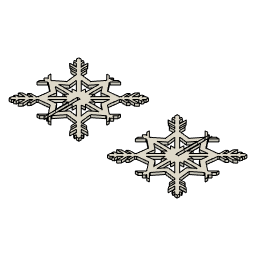
fulg (Autodesk Fusion 360 design; units mm, degrees)
Autodesk Fusion 360 part; units mm, degrees
sketch "Sketch1" plane through (0, 0, 0) normal (0, 1, 0) x (1, 0, 0)
  line L0 (40, 40) -> (-40, 40) construction
  line L1 (-40, 40) -> (-40, -40) construction
  line L2 (-40, -40) -> (40, -40) construction
  line L3 (40, -40) -> (40, 40) construction
  line L4 (40, 40) -> (-40, -40) construction
  dimension "d1" = 80
  dimension "d2" = 80
  constraint perpendicular L0 L1
  constraint parallel L0 L2
  constraint parallel L1 L3
  constraint horizontal L0
  constraint coincident L4 origin
  measures "d1" distance of L1.end L2.end
  measures "d2" distance of L0.end L1.end
sketch "Sketch3" plane through (0, 0, 0) normal (0, 1, 0) x (1, 0, 0)
  line L0 (0, 40) -> (0, 35) construction
  line L1 (40, 0) -> (46.0201, 0) construction
  line L2 (-40, 0) -> (-46.178, 0) construction
  line L3 (0.0024, 40) -> (-0.0024, 40)
  arc A0 (0.0024, 40) -> (-0.0024, 40) centre (0, 37.5) ccw
  line L4 (-40, 40) -> (-40, 37.1716)
  line L5 (-40, 40) -> (-37.1716, 40)
  line L6 (40, -40) -> (40, -37.1716)
  line L7 (40, -37.1716) -> (40, -40)
  line L8 (37.1716, -40) -> (40, -40)
  line L9 (-40, -40) -> (-38, -40) construction
  line L10 (-40, -40) -> (-40, -37.1716)
  line L11 (-40, -40) -> (-37.1716, -40)
  line L12 (40, 40) -> (40, 37.1716)
  line L13 (40, 40) -> (37.1716, 40)
  line L14 (-5.3576, 12.9343) -> (-5.514, 8.3424)
  line L15 (-5.3576, 12.9343) -> (-2, 9.798)
  line L16 (12.9343, -5.3576) -> (8.3424, -5.514)
  line L17 (12.9343, -5.3576) -> (9.798, -2)
  line L18 (5.3576, 12.9343) -> (5.514, 8.3424)
  line L19 (5.3576, 12.9343) -> (2, 9.798)
  line L20 (-5.3576, -12.9343) -> (-5.514, -8.3424)
  line L21 (-5.3576, -12.9343) -> (-2, -9.798)
  line L22 (-12.9343, 5.3576) -> (-8.3424, 5.514)
  line L23 (-12.9343, 5.3576) -> (-9.798, 2)
  line L24 (-12.9343, -5.3576) -> (-9.798, -2)
  line L25 (-12.9343, -5.3576) -> (-8.3424, -5.514)
  line L26 (5.3576, -12.9343) -> (5.514, -8.3424)
  line L27 (5.3576, -12.9343) -> (2, -9.798)
  line L28 (12.9343, 5.3576) -> (9.798, 2)
  line L29 (12.9343, 5.3576) -> (8.3424, 5.514)
  line L30 (-16.2068, 19.0352) -> (-5.514, 8.3424)
  line L31 (-7.4559, 17.9962) -> (-2, 24.899)
  line L32 (-2, 24.899) -> (-2, 9.798)
  line L33 (-7.4559, 17.9962) -> (-16.2068, 19.0352)
  line L34 (-19.0352, 16.2068) -> (-8.3424, 5.514)
  line L35 (-24.899, -2) -> (-9.798, -2)
  line L36 (-8.3424, -5.514) -> (-19.0352, -16.2068)
  line L37 (-16.2068, -19.0352) -> (-5.514, -8.3424)
  line L38 (-2, -9.798) -> (-2, -24.899)
  line L39 (2, -24.899) -> (2, -9.798)
  line L40 (5.514, -8.3424) -> (16.2068, -19.0352)
  line L41 (19.0352, -16.2068) -> (8.3424, -5.514)
  line L42 (9.798, -2) -> (24.899, -2)
  line L43 (24.899, 2) -> (9.798, 2)
  line L44 (8.3424, 5.514) -> (19.0352, 16.2068)
  line L45 (16.2068, 19.0352) -> (5.514, 8.3424)
  line L46 (2, 24.899) -> (2, 9.798)
  line L47 (7.4559, 17.9962) -> (16.2068, 19.0352)
  line L48 (7.4559, 17.9962) -> (2, 24.899)
  line L49 (17.9962, 7.4559) -> (24.899, 2)
  line L50 (17.9962, 7.4559) -> (19.0352, 16.2068)
  line L51 (17.9962, -7.4559) -> (19.0352, -16.2068)
  line L52 (24.899, -2) -> (17.9962, -7.4559)
  line L53 (7.4559, -17.9962) -> (2, -24.899)
  line L54 (7.4559, -17.9962) -> (16.2068, -19.0352)
  line L55 (-7.4559, -17.9962) -> (-16.2068, -19.0352)
  line L56 (-7.4559, -17.9962) -> (-2, -24.899)
  line L57 (-17.9962, -7.4559) -> (-24.899, -2)
  line L58 (-17.9962, -7.4559) -> (-19.0352, -16.2068)
  line L59 (-17.9962, 7.4559) -> (-19.0352, 16.2068)
  line L60 (-17.9962, 7.4559) -> (-24.899, 2)
  line L61 (-23.2912, 9.644) -> (-27.9994, 5.9227)
  line L62 (-23.2912, 9.644) -> (-24.0004, 15.6173)
  line L63 (-24.0004, 15.6173) -> (-24.7487, 21.9203)
  line L64 (-23.2912, 9.644) -> (-32.9624, 2)
  line L65 (-24.9199, 2) -> (-9.798, 2)
  line L66 (23.2912, 9.644) -> (32.9624, 2)
  line L67 (23.2912, 9.644) -> (24.7487, 21.9203)
  line L68 (19.0352, 16.2068) -> (8.3424, 5.514)
  line L69 (9.798, 2) -> (24.9199, 2)
  line L70 (23.2912, -9.644) -> (24.0004, -15.6173)
  line L71 (32.9624, -2) -> (23.2912, -9.644)
  line L72 (23.2912, -9.644) -> (24.7487, -21.9203)
  line L73 (9.644, -23.2912) -> (15.6173, -24.0004)
  line L74 (9.644, -23.2912) -> (2, -32.9624)
  line L75 (9.644, -23.2912) -> (21.9203, -24.7487)
  line L76 (7, -9.8284) -> (7, -9.798)
  line L77 (-9.644, -23.2912) -> (-7, -26.6364)
  line L78 (-9.644, -23.2912) -> (-15.6173, -24.0004)
  line L79 (-9.644, -23.2912) -> (-2, -32.9624)
  line L80 (-9.644, -23.2912) -> (-21.9203, -24.7487)
  line L81 (-23.2912, -9.644) -> (-26.6364, -7)
  line L82 (-23.2912, -9.644) -> (-24.0004, -15.6173)
  line L83 (-23.2912, -9.644) -> (-32.9624, -2)
  line L84 (-23.2912, -9.644) -> (-24.7487, -21.9203)
  line L85 (3, 10.7321) -> (3, 9.798)
  line L86 (-9.644, 23.2912) -> (-15.6173, 24.0004)
  line L87 (-9.644, 23.2912) -> (-2, 32.9624)
  line L88 (-9.644, 23.2912) -> (-21.9203, 24.7487)
  line L89 (9.644, 23.2912) -> (15.6173, 24.0004)
  line L90 (9.644, 23.2912) -> (7, 26.6364)
  line L91 (-7, 9.8284) -> (-7, 9.798)
  line L92 (9.644, 23.2912) -> (2, 32.9624)
  line L93 (9.644, 23.2912) -> (21.9203, 24.7487)
  line L94 (5.514, 8.3424) -> (16.2068, 19.0352)
  line L95 (2, 9.798) -> (2, 24.9199)
  line L96 (-2, 24.9199) -> (-2, 9.798)
  line L97 (-5.514, 8.3424) -> (-16.2068, 19.0352)
  line L98 (-9.798, -2) -> (-24.9199, -2)
  line L99 (-5.514, -8.3424) -> (-16.2068, -19.0352)
  line L100 (-2, -9.798) -> (-2, -24.9199)
  line L101 (2, -24.9199) -> (2, -9.798)
  line L102 (5.514, -8.3424) -> (16.2068, -19.0352)
  line L103 (19.0352, -16.2068) -> (8.3424, -5.514)
  line L104 (24.9199, -2) -> (9.798, -2)
  line L105 (-40, 0) -> (-38, 2)
  line L106 (-40, 0) -> (-38, -2)
  line L107 (-34, 2) -> (-40, 8)
  line L108 (-37, 2) -> (-40, 5)
  line L109 (-40, 5) -> (-40, 8)
  line L110 (-37, -2) -> (-40, -5)
  line L111 (-40, -5) -> (-40, -8)
  line L112 (-40, -8) -> (-34, -2)
  line L113 (-38, 2) -> (-37, 2)
  line L114 (-34, 2) -> (-32.9624, 2)
  line L115 (-32.9624, -2) -> (-34, -2)
  line L116 (-37, -2) -> (-38, -2)
  line L117 (40, 0) -> (37.9962, 2)
  line L118 (40, 0) -> (38.0038, -2)
  line L119 (37.0369, 2) -> (40, 4.9687)
  line L120 (40, 4.9687) -> (40, 7.9488)
  line L121 (40, 7.9488) -> (34.0625, 2)
  line L122 (37.0369, -2) -> (40, -4.9575)
  line L123 (40, -4.9575) -> (40, -8)
  line L124 (40, -8) -> (33.9886, -2)
  line L125 (32.9624, 2) -> (34.0625, 2)
  line L126 (37.0369, 2) -> (37.9962, 2)
  line L127 (38.0038, -2) -> (37.0369, -2)
  line L128 (33.9886, -2) -> (32.9624, -2)
  line L129 (0, -40) -> (2, -38)
  line L130 (0, -40) -> (-2, -38)
  line L131 (-2, -36.9976) -> (-5.0024, -40)
  line L132 (-5.0024, -40) -> (-7.9912, -40)
  line L133 (-7.9912, -40) -> (-2, -34.0088)
  line L134 (2, -34.0088) -> (7.9912, -40)
  line L135 (7.9912, -40) -> (4.9956, -40)
  line L136 (4.9956, -40) -> (2, -37.0044)
  line L137 (2, -38) -> (2, -37.0044)
  line L138 (2, -34.0088) -> (2, -32.9624)
  line L139 (-2, -32.9624) -> (-2, -34.0088)
  line L140 (-2, -36.9976) -> (-2, -38)
  line L141 (-0.0024, 40) -> (2, 38)
  line L142 (-0.0024, 40) -> (-2, 38)
  line L143 (-2, 36.9767) -> (-5.027, 40)
  line L144 (-5.027, 40) -> (-7.9448, 40)
  line L145 (-7.9448, 40) -> (-2, 34.0624)
  line L146 (2, 37) -> (4.9963, 40)
  line L147 (4.9963, 40) -> (8, 40)
  line L148 (8, 40) -> (2, 33.9927)
  line L149 (2, 32.9624) -> (2, 33.9927)
  line L150 (2, 37) -> (2, 38)
  line L151 (-2, 38) -> (-2, 36.9767)
  line L152 (-2, 34.0624) -> (-2, 32.9624)
  line L153 (-35.01, 37.8385) -> (-35.01, 40)
  line L154 (-35.01, 40) -> (-32.9636, 38.9192)
  line L155 (-32.9636, 38.9192) -> (-32.9636, 35.792)
  line L156 (-37.8689, 35.0405) -> (-40, 35.0405)
  line L157 (-40, 35.0405) -> (-38.9345, 32.942)
  line L158 (-38.9345, 32.942) -> (-35.7705, 32.942)
  line L159 (-29.5459, 32.3743) -> (-29.5459, 40)
  line L160 (-29.5459, 40) -> (-27, 37)
  line L161 (-27, 37) -> (-27, 29.8284)
  line L162 (-32.3743, 29.5459) -> (-40, 29.5459)
  line L163 (-40, 29.5459) -> (-37, 27)
  line L164 (-37, 27) -> (-29.8284, 27)
  line L165 (-22.999, 25.8274) -> (-22.999, 32)
  line L166 (-22.999, 32) -> (-24.9897, 33.9907)
  line L167 (-24.9897, 33.9907) -> (-24.9897, 27.8181)
  line L168 (-25.7878, 22.9594) -> (-32, 22.9594)
  line L169 (-32, 22.9594) -> (-34.0154, 24.9748)
  line L170 (-34.0154, 24.9748) -> (-27.8032, 24.9748)
  line L171 (-40, 37.1716) -> (-37.8689, 35.0405)
  line L172 (-35.01, 37.8385) -> (-37.1716, 40)
  line L173 (-29.5459, 32.3743) -> (-32.9636, 35.792)
  line L174 (-21.9203, 24.7487) -> (-22.999, 25.8274)
  line L175 (-24.9897, 27.8181) -> (-27, 29.8284)
  line L176 (-25.7878, 22.9594) -> (-24.7487, 21.9203)
  line L177 (-35.7705, 32.942) -> (-32.3743, 29.5459)
  line L178 (-29.8284, 27) -> (-27.8032, 24.9748)
  line L179 (35.01, 37.8385) -> (35.01, 40)
  line L180 (35.01, 40) -> (32.9636, 38.9192)
  line L181 (32.9636, 38.9192) -> (32.9636, 35.792)
  line L182 (37.8689, 35.0405) -> (40, 35.0405)
  line L183 (40, 35.0405) -> (38.9345, 32.942)
  line L184 (38.9345, 32.942) -> (35.7705, 32.942)
  line L185 (32.3743, 29.5459) -> (40, 29.5459)
  line L186 (40, 29.5459) -> (37, 27)
  line L187 (37, 27) -> (29.8284, 27)
  line L188 (34.0154, 24.9748) -> (27.8032, 24.9748)
  line L189 (32, 22.9594) -> (34.0154, 24.9748)
  line L190 (25.7878, 22.9594) -> (32, 22.9594)
  line L191 (24.9897, 33.9907) -> (24.9897, 27.8181)
  line L192 (22.999, 32) -> (24.9897, 33.9907)
  line L193 (22.999, 25.8274) -> (22.999, 32)
  line L194 (27, 37) -> (27, 29.8284)
  line L195 (29.5459, 40) -> (27, 37)
  line L196 (29.5459, 32.3743) -> (29.5459, 40)
  line L197 (32.9636, -38.9192) -> (32.9636, -35.792)
  line L198 (35.01, -40) -> (32.9636, -38.9192)
  line L199 (35.01, -37.8385) -> (35.01, -40)
  line L200 (29.5459, -32.3743) -> (29.5459, -40)
  line L201 (29.5459, -40) -> (27, -37)
  line L202 (27, -37) -> (27, -29.8284)
  line L203 (24.9897, -33.9907) -> (24.9897, -27.8181)
  line L204 (22.999, -32) -> (24.9897, -33.9907)
  line L205 (22.999, -25.8274) -> (22.999, -32)
  line L206 (34.0154, -24.9748) -> (27.8032, -24.9748)
  line L207 (25.7878, -22.9594) -> (32, -22.9594)
  line L208 (32, -22.9594) -> (34.0154, -24.9748)
  line L209 (37, -27) -> (29.8284, -27)
  line L210 (40, -29.5459) -> (37, -27)
  line L211 (32.3743, -29.5459) -> (40, -29.5459)
  line L212 (38.9345, -32.942) -> (35.7705, -32.942)
  line L213 (40, -35.0405) -> (38.9345, -32.942)
  line L214 (37.8689, -35.0405) -> (40, -35.0405)
  line L215 (-22.999, -25.8274) -> (-22.999, -32)
  line L216 (-22.999, -32) -> (-24.9897, -33.9907)
  line L217 (-24.9897, -33.9907) -> (-24.9897, -27.8181)
  line L218 (-27, -37) -> (-27, -29.8284)
  line L219 (-29.5459, -40) -> (-27, -37)
  line L220 (-29.5459, -32.3743) -> (-29.5459, -40)
  line L221 (-32.9636, -38.9192) -> (-32.9636, -35.792)
  line L222 (-35.01, -40) -> (-32.9636, -38.9192)
  line L223 (-35.01, -37.8385) -> (-35.01, -40)
  line L224 (-37.8689, -35.0405) -> (-40, -35.0405)
  line L225 (-40, -35.0405) -> (-38.9345, -32.942)
  line L226 (-38.9345, -32.942) -> (-35.7705, -32.942)
  line L227 (-32.3743, -29.5459) -> (-40, -29.5459)
  line L228 (-40, -29.5459) -> (-37, -27)
  line L229 (-37, -27) -> (-29.8284, -27)
  line L230 (-34.0154, -24.9748) -> (-27.8032, -24.9748)
  line L231 (-32, -22.9594) -> (-34.0154, -24.9748)
  line L232 (-25.7878, -22.9594) -> (-32, -22.9594)
  line L233 (-25.7878, -22.9594) -> (-24.7487, -21.9203)
  line L234 (-29.8284, -27) -> (-27.8032, -24.9748)
  line L235 (-40, -37.1716) -> (-37.8689, -35.0405)
  line L236 (-35.7705, -32.942) -> (-32.3743, -29.5459)
  line L237 (-35.01, -37.8385) -> (-37.1716, -40)
  line L238 (-29.5459, -32.3743) -> (-32.9636, -35.792)
  line L239 (-21.9203, -24.7487) -> (-22.999, -25.8274)
  line L240 (-24.9897, -27.8181) -> (-27, -29.8284)
  line L241 (21.9203, -24.7487) -> (22.999, -25.8274)
  line L242 (24.9897, -27.8181) -> (27, -29.8284)
  line L243 (29.5459, -32.3743) -> (32.9636, -35.792)
  line L244 (35.01, -37.8385) -> (37.1716, -40)
  line L245 (40, -37.1716) -> (37.8689, -35.0405)
  line L246 (35.7705, -32.942) -> (32.3743, -29.5459)
  line L247 (29.8284, -27) -> (27.8032, -24.9748)
  line L248 (25.7878, -22.9594) -> (24.7487, -21.9203)
  line L249 (35.01, 37.8385) -> (37.1716, 40)
  line L250 (29.5459, 32.3743) -> (32.9636, 35.792)
  line L251 (21.9203, 24.7487) -> (22.999, 25.8274)
  line L252 (24.9897, 27.8181) -> (27, 29.8284)
  line L253 (25.7878, 22.9594) -> (24.7487, 21.9203)
  line L254 (29.8284, 27) -> (27.8032, 24.9748)
  line L255 (40, 37.1716) -> (37.8689, 35.0405)
  line L256 (35.7705, 32.942) -> (32.3743, 29.5459)
  dimension "d20" = 5
  constraint vertical L0
  constraint midpoint L0 A0.centre
  constraint coincident L0.start A0
  constraint horizontal L1
  constraint horizontal L2
  constraint perpendicular L3 L137
  constraint vertical L4
  constraint perpendicular L4 L5
  constraint perpendicular L5 L6
  constraint parallel L6 L7
  constraint perpendicular L7 L8
  constraint horizontal L9
  constraint perpendicular L9 L10
  constraint perpendicular L10 L11
  constraint perpendicular L12 L113
  constraint perpendicular L12 L13
  constraint collinear L97 L245
  constraint collinear L94 L235
  constraint collinear L98 L127
  constraint collinear L99 L255
  constraint symmetric L2 L22.start L24.start
  constraint symmetric L2 L22.end L25.end
  constraint symmetric L2 L23.end L24.end
  constraint parallel L30 L97
  constraint parallel L34 L171
  constraint parallel L36 L235
  constraint parallel L37 L99
  constraint parallel L38 L100
  constraint parallel L40 L102
  constraint coincident L41.start L245
  constraint parallel L41 L245
  constraint coincident L44.end L255
  constraint parallel L44 L255
  constraint parallel L45 L94
  constraint parallel L46 L95
  constraint coincident L65.start L113
  constraint coincident L96.start L151
  constraint coincident L104.start L127
  constraint coincident L101.start L137
  constraint parallel L62 L63
  constraint parallel L61 L64
  constraint collinear L65 L113
  constraint coincident L60.end L113
  constraint parallel L50 L67
  constraint parallel L49 L66
  constraint coincident L66.end L69
  constraint collinear L68 L255
  constraint collinear L69 L125
  constraint coincident L43.start L69
  constraint parallel L51 L70
  constraint parallel L52 L71
  constraint parallel L70 L72
  constraint parallel L54 L73
  constraint parallel L53 L74
  constraint coincident L75.end L102
  constraint parallel L73 L75
  constraint parallel L76 L137
  constraint parallel L56 L77
  constraint parallel L55 L78
  constraint coincident L76.start L102
  constraint coincident L79.end L100
  constraint parallel L77 L79
  constraint coincident L80.end L99
  constraint parallel L78 L80
  constraint parallel L57 L81
  constraint parallel L58 L82
  constraint coincident L83.end L98
  constraint parallel L81 L83
  constraint parallel L82 L84
  constraint parallel L32 L85
  constraint parallel L31 L87
  constraint parallel L33 L86
  constraint coincident L19 L85.start
  constraint coincident L88.end L97
  constraint parallel L86 L88
  constraint parallel L47 L89
  constraint parallel L48 L90
  constraint parallel L91 L151
  constraint coincident L91.start L97
  constraint coincident L92.end L95
  constraint parallel L90 L92
  constraint coincident L93.end L94
  constraint parallel L89 L93
  constraint collinear L94 L251
  constraint collinear L95 L149
  constraint coincident L46.start L95
  constraint collinear L96 L151
  constraint coincident L31.end L151
  constraint collinear L97 L174
  constraint collinear L98 L115
  constraint coincident L35.start L98
  constraint collinear L99 L239
  constraint collinear L100 L139
  constraint coincident L38.end L100
  constraint collinear L101 L137
  constraint coincident L39.start L137
  constraint collinear L102 L241
  constraint collinear L103 L245
  constraint collinear L104 L127
  constraint coincident L42.end L127
  constraint perpendicular L105 L106
  constraint coincident L107.start L113
  constraint perpendicular L109 L113
  constraint coincident L110.start L115
  constraint perpendicular L107 L110
  constraint perpendicular L111 L115
  constraint perpendicular L107 L112
  constraint collinear L113 L114
  constraint collinear L115 L116
  constraint coincident L117.end L125
  constraint perpendicular L117 L118
  constraint coincident L119.start L125
  constraint perpendicular L117 L119
  constraint perpendicular L120 L125
  constraint perpendicular L117 L121
  constraint perpendicular L121 L122
  constraint perpendicular L123 L127
  constraint coincident L124.end L127
  constraint parallel L122 L124
  constraint collinear L125 L126
  constraint collinear L127 L128
  constraint perpendicular L129 L130
  constraint coincident L131.start L139
  constraint perpendicular L130 L131
  constraint perpendicular L132 L139
  constraint perpendicular L130 L133
  constraint coincident L134.start L137
  constraint perpendicular L133 L134
  constraint perpendicular L135 L137
  constraint parallel L134 L136
  constraint collinear L137 L138
  constraint collinear L139 L140
  constraint perpendicular L141 L142
  constraint perpendicular L142 L143
  constraint perpendicular L144 L151
  constraint coincident L145.end L151
  constraint perpendicular L142 L145
  constraint coincident L146.start L149
  constraint perpendicular L145 L146
  constraint perpendicular L147 L149
  constraint perpendicular L145 L148
  constraint collinear L149 L150
  constraint collinear L151 L152
  constraint coincident L153.start L174
  constraint vertical L153
  constraint parallel L153 L155
  constraint perpendicular L155 L156
  constraint coincident L158.end L171
  constraint parallel L156 L158
  constraint vertical L159
  constraint parallel L159 L161
  constraint perpendicular L161 L162
  constraint coincident L164.end L171
  constraint perpendicular L161 L164
  constraint vertical L165
  constraint parallel L166 L174
  constraint coincident L167.end L174
  constraint parallel L165 L167
  constraint coincident L168.start L171
  constraint perpendicular L167 L168
  constraint parallel L169 L171
  constraint coincident L170.end L171
  constraint parallel L168 L170
  constraint collinear L171 L177
  constraint coincident L162.start L171
  constraint collinear L172 L174
  constraint coincident L159.start L174
  constraint collinear L173 L174
  constraint collinear L174 L175
  constraint collinear L176 L177
  constraint collinear L177 L178
  constraint collinear L233 L235
  constraint collinear L234 L235
  constraint collinear L235 L236
  constraint collinear L237 L239
  constraint collinear L238 L239
  constraint collinear L239 L240
  constraint collinear L241 L242
  constraint collinear L242 L243
  constraint collinear L243 L244
  constraint collinear L245 L246
  constraint collinear L246 L247
  constraint collinear L247 L248
  constraint collinear L249 L251
  constraint collinear L250 L251
  constraint collinear L251 L252
  constraint collinear L253 L255
  constraint collinear L254 L255
  constraint collinear L255 L256
extrude "Extrude1" add sketch "Sketch3" along normal blind 3 makes body 1
sketch "Sketch4" plane through (0, 3, 0) normal (0, 1, 0) x (-1, 0, 0)
  line L0 (-8.3424, 5.514) -> (-12.9343, 5.3576)
  line L1 (-12.9343, 5.3576) -> (-9.798, 2)
  line L2 (-9.798, 2) -> (-24.899, 2)
  line L3 (-24.899, 2) -> (-17.9962, 7.4559)
  line L4 (-17.9962, 7.4559) -> (-19.0352, 16.2068)
  line L5 (-19.0352, 16.2068) -> (-8.3424, 5.514)
  line L6 (5.514, 8.3424) -> (5.3576, 12.9343)
  line L7 (5.3576, 12.9343) -> (2, 9.798)
  line L8 (2, 9.798) -> (2, 24.899)
  line L9 (2, 24.899) -> (7.4559, 17.9962)
  line L10 (7.4559, 17.9962) -> (16.2068, 19.0352)
  line L11 (16.2068, 19.0352) -> (5.514, 8.3424)
  line L12 (-2, 9.798) -> (-5.3576, 12.9343)
  line L13 (-5.3576, 12.9343) -> (-5.514, 8.3424)
  line L14 (-5.514, 8.3424) -> (-16.2068, 19.0352)
  line L15 (-16.2068, 19.0352) -> (-7.4559, 17.9962)
  line L16 (-7.4559, 17.9962) -> (-2, 24.899)
  line L17 (-2, 24.899) -> (-2, 9.798)
  line L18 (2, -9.798) -> (5.3576, -12.9343)
  line L19 (5.3576, -12.9343) -> (5.514, -8.3424)
  line L20 (5.514, -8.3424) -> (16.2068, -19.0352)
  line L21 (16.2068, -19.0352) -> (7.4559, -17.9962)
  line L22 (7.4559, -17.9962) -> (2, -24.899)
  line L23 (2, -24.899) -> (2, -9.798)
  line L24 (9.798, 2) -> (12.9343, 5.3576)
  line L25 (12.9343, 5.3576) -> (8.3424, 5.514)
  line L26 (8.3424, 5.514) -> (19.0352, 16.2068)
  line L27 (19.0352, 16.2068) -> (17.9962, 7.4559)
  line L28 (17.9962, 7.4559) -> (24.899, 2)
  line L29 (24.899, 2) -> (9.798, 2)
  line L30 (-5.514, -8.3424) -> (-5.3576, -12.9343)
  line L31 (-5.3576, -12.9343) -> (-2, -9.798)
  line L32 (-2, -9.798) -> (-2, -24.899)
  line L33 (-2, -24.899) -> (-7.4559, -17.9962)
  line L34 (-7.4559, -17.9962) -> (-16.2068, -19.0352)
  line L35 (-16.2068, -19.0352) -> (-5.514, -8.3424)
  line L36 (-9.798, -2) -> (-12.9343, -5.3576)
  line L37 (-12.9343, -5.3576) -> (-8.3424, -5.514)
  line L38 (-8.3424, -5.514) -> (-19.0352, -16.2068)
  line L39 (-19.0352, -16.2068) -> (-17.9962, -7.4559)
  line L40 (-17.9962, -7.4559) -> (-24.899, -2)
  line L41 (-24.899, -2) -> (-9.798, -2)
  line L42 (17.9962, -7.4559) -> (19.0352, -16.2068)
  line L43 (19.0352, -16.2068) -> (8.3424, -5.514)
  line L44 (8.3424, -5.514) -> (12.9343, -5.3576)
  line L45 (12.9343, -5.3576) -> (9.798, -2)
  line L46 (9.798, -2) -> (24.899, -2)
  line L47 (24.899, -2) -> (17.9962, -7.4559)
  line L48 (-40, -40) -> (-37.1716, -40)
  line L49 (-37.1716, -40) -> (-35.01, -37.8385)
  line L50 (-35.01, -37.8385) -> (-35.01, -40)
  line L51 (-35.01, -40) -> (-32.9636, -38.9192)
  line L52 (-32.9636, -38.9192) -> (-32.9636, -35.792)
  line L53 (-32.9636, -35.792) -> (-29.5459, -32.3743)
  line L54 (-29.5459, -32.3743) -> (-29.5459, -40)
  line L55 (-29.5459, -40) -> (-27, -37)
  line L56 (-27, -37) -> (-27, -29.8284)
  line L57 (-27, -29.8284) -> (-24.9897, -27.8181)
  line L58 (-24.9897, -27.8181) -> (-24.9897, -33.9907)
  line L59 (-24.9897, -33.9907) -> (-22.999, -32)
  line L60 (-22.999, -32) -> (-22.999, -25.8274)
  line L61 (-22.999, -25.8274) -> (-21.9203, -24.7487)
  line L62 (-21.9203, -24.7487) -> (-9.644, -23.2912)
  line L63 (-9.644, -23.2912) -> (-2, -32.9624)
  line L64 (-2, -32.9624) -> (-2, -33.9927)
  line L65 (-2, -33.9927) -> (-8, -40)
  line L66 (-8, -40) -> (-4.9963, -40)
  line L67 (-4.9963, -40) -> (-2, -37)
  line L68 (-2, -37) -> (-2, -38)
  line L69 (-2, -38) -> (0.0024, -40)
  line L70 (0.0024, -40) -> (2, -38)
  line L71 (2, -38) -> (2, -36.9767)
  line L72 (2, -36.9767) -> (5.027, -40)
  line L73 (5.027, -40) -> (7.9448, -40)
  line L74 (7.9448, -40) -> (2, -34.0624)
  line L75 (2, -34.0624) -> (2, -32.9624)
  line L76 (2, -32.9624) -> (9.644, -23.2912)
  line L77 (9.644, -23.2912) -> (21.9203, -24.7487)
  line L78 (21.9203, -24.7487) -> (22.999, -25.8274)
  line L79 (22.999, -25.8274) -> (22.999, -32)
  line L80 (22.999, -32) -> (24.9897, -33.9907)
  line L81 (24.9897, -33.9907) -> (24.9897, -27.8181)
  line L82 (24.9897, -27.8181) -> (27, -29.8284)
  line L83 (27, -29.8284) -> (27, -37)
  line L84 (27, -37) -> (29.5459, -40)
  line L85 (29.5459, -40) -> (29.5459, -32.3743)
  line L86 (29.5459, -32.3743) -> (32.9636, -35.792)
  line L87 (32.9636, -35.792) -> (32.9636, -38.9192)
  line L88 (32.9636, -38.9192) -> (35.01, -40)
  line L89 (35.01, -40) -> (35.01, -37.8385)
  line L90 (35.01, -37.8385) -> (37.1716, -40)
  line L91 (37.1716, -40) -> (40, -40)
  line L92 (40, -40) -> (40, -37.1716)
  line L93 (40, -37.1716) -> (37.8689, -35.0405)
  line L94 (37.8689, -35.0405) -> (40, -35.0405)
  line L95 (40, -35.0405) -> (38.9345, -32.942)
  line L96 (38.9345, -32.942) -> (35.7705, -32.942)
  line L97 (35.7705, -32.942) -> (32.3743, -29.5459)
  line L98 (32.3743, -29.5459) -> (40, -29.5459)
  line L99 (40, -29.5459) -> (37, -27)
  line L100 (37, -27) -> (29.8284, -27)
  line L101 (29.8284, -27) -> (27.8032, -24.9748)
  line L102 (27.8032, -24.9748) -> (34.0154, -24.9748)
  line L103 (34.0154, -24.9748) -> (32, -22.9594)
  line L104 (32, -22.9594) -> (25.7878, -22.9594)
  line L105 (25.7878, -22.9594) -> (24.7487, -21.9203)
  line L106 (24.7487, -21.9203) -> (23.2912, -9.644)
  line L107 (23.2912, -9.644) -> (32.9624, -2)
  line L108 (32.9624, -2) -> (34, -2)
  line L109 (34, -2) -> (40, -8)
  line L110 (40, -8) -> (40, -5)
  line L111 (40, -5) -> (37, -2)
  line L112 (37, -2) -> (38, -2)
  line L113 (38, -2) -> (40, 0)
  line L114 (40, 0) -> (38, 2)
  line L115 (38, 2) -> (37, 2)
  line L116 (37, 2) -> (40, 5)
  line L117 (40, 5) -> (40, 8)
  line L118 (40, 8) -> (34, 2)
  line L119 (34, 2) -> (32.9624, 2)
  line L120 (32.9624, 2) -> (23.2912, 9.644)
  line L121 (23.2912, 9.644) -> (24.7487, 21.9203)
  line L122 (24.7487, 21.9203) -> (25.7878, 22.9594)
  line L123 (25.7878, 22.9594) -> (32, 22.9594)
  line L124 (32, 22.9594) -> (34.0154, 24.9748)
  line L125 (34.0154, 24.9748) -> (27.8032, 24.9748)
  line L126 (27.8032, 24.9748) -> (29.8284, 27)
  line L127 (29.8284, 27) -> (37, 27)
  line L128 (37, 27) -> (40, 29.5459)
  line L129 (40, 29.5459) -> (32.3743, 29.5459)
  line L130 (32.3743, 29.5459) -> (35.7705, 32.942)
  line L131 (35.7705, 32.942) -> (38.9345, 32.942)
  line L132 (38.9345, 32.942) -> (40, 35.0405)
  line L133 (40, 35.0405) -> (37.8689, 35.0405)
  line L134 (37.8689, 35.0405) -> (40, 37.1716)
  line L135 (40, 37.1716) -> (40, 40)
  line L136 (40, 40) -> (37.1716, 40)
  line L137 (37.1716, 40) -> (35.01, 37.8385)
  line L138 (35.01, 37.8385) -> (35.01, 40)
  line L139 (35.01, 40) -> (32.9636, 38.9192)
  line L140 (32.9636, 38.9192) -> (32.9636, 35.792)
  line L141 (32.9636, 35.792) -> (29.5459, 32.3743)
  line L142 (29.5459, 32.3743) -> (29.5459, 40)
  line L143 (29.5459, 40) -> (27, 37)
  line L144 (27, 37) -> (27, 29.8284)
  line L145 (27, 29.8284) -> (24.9897, 27.8181)
  line L146 (24.9897, 27.8181) -> (24.9897, 33.9907)
  line L147 (24.9897, 33.9907) -> (22.999, 32)
  line L148 (22.999, 32) -> (22.999, 25.8274)
  line L149 (22.999, 25.8274) -> (21.9203, 24.7487)
  line L150 (21.9203, 24.7487) -> (9.644, 23.2912)
  line L151 (9.644, 23.2912) -> (2, 32.9624)
  line L152 (2, 32.9624) -> (2, 34.0088)
  line L153 (2, 34.0088) -> (7.9912, 40)
  line L154 (7.9912, 40) -> (5.0024, 40)
  line L155 (5.0024, 40) -> (2, 36.9976)
  line L156 (2, 36.9976) -> (2, 38)
  line L157 (2, 38) -> (0, 40)
  line L158 (0, 40) -> (-2, 38)
  line L159 (-2, 38) -> (-2, 37.0044)
  line L160 (-2, 37.0044) -> (-4.9956, 40)
  line L161 (-4.9956, 40) -> (-7.9912, 40)
  line L162 (-7.9912, 40) -> (-2, 34.0088)
  line L163 (-2, 34.0088) -> (-2, 32.9624)
  line L164 (-2, 32.9624) -> (-9.644, 23.2912)
  line L165 (-9.644, 23.2912) -> (-21.9203, 24.7487)
  line L166 (-21.9203, 24.7487) -> (-22.999, 25.8274)
  line L167 (-22.999, 25.8274) -> (-22.999, 32)
  line L168 (-22.999, 32) -> (-24.9897, 33.9907)
  line L169 (-24.9897, 33.9907) -> (-24.9897, 27.8181)
  line L170 (-24.9897, 27.8181) -> (-27, 29.8284)
  line L171 (-27, 29.8284) -> (-27, 37)
  line L172 (-27, 37) -> (-29.5459, 40)
  line L173 (-29.5459, 40) -> (-29.5459, 32.3743)
  line L174 (-29.5459, 32.3743) -> (-32.9636, 35.792)
  line L175 (-32.9636, 35.792) -> (-32.9636, 38.9192)
  line L176 (-32.9636, 38.9192) -> (-35.01, 40)
  line L177 (-35.01, 40) -> (-35.01, 37.8385)
  line L178 (-35.01, 37.8385) -> (-37.1716, 40)
  line L179 (-37.1716, 40) -> (-40, 40)
  line L180 (-40, 40) -> (-40, 37.1716)
  line L181 (-40, 37.1716) -> (-37.8689, 35.0405)
  line L182 (-37.8689, 35.0405) -> (-40, 35.0405)
  line L183 (-40, 35.0405) -> (-38.9345, 32.942)
  line L184 (-38.9345, 32.942) -> (-35.7705, 32.942)
  line L185 (-35.7705, 32.942) -> (-32.3743, 29.5459)
  line L186 (-32.3743, 29.5459) -> (-40, 29.5459)
  line L187 (-40, 29.5459) -> (-37, 27)
  line L188 (-37, 27) -> (-29.8284, 27)
  line L189 (-29.8284, 27) -> (-27.8032, 24.9748)
  line L190 (-27.8032, 24.9748) -> (-34.0154, 24.9748)
  line L191 (-34.0154, 24.9748) -> (-32, 22.9594)
  line L192 (-32, 22.9594) -> (-25.7878, 22.9594)
  line L193 (-25.7878, 22.9594) -> (-24.7487, 21.9203)
  line L194 (-24.7487, 21.9203) -> (-23.2912, 9.644)
  line L195 (-23.2912, 9.644) -> (-32.9624, 2)
  line L196 (-32.9624, 2) -> (-33.9886, 2)
  line L197 (-33.9886, 2) -> (-40, 8)
  line L198 (-40, 8) -> (-40, 4.9575)
  line L199 (-40, 4.9575) -> (-37.0369, 2)
  line L200 (-37.0369, 2) -> (-38.0038, 2)
  line L201 (-38.0038, 2) -> (-40, 0)
  line L202 (-40, 0) -> (-37.9962, -2)
  line L203 (-37.9962, -2) -> (-37.0369, -2)
  line L204 (-37.0369, -2) -> (-40, -4.9687)
  line L205 (-40, -4.9687) -> (-40, -7.9488)
  line L206 (-40, -7.9488) -> (-34.0625, -2)
  line L207 (-34.0625, -2) -> (-32.9624, -2)
  line L208 (-32.9624, -2) -> (-23.2912, -9.644)
  line L209 (-23.2912, -9.644) -> (-24.7487, -21.9203)
  line L210 (-24.7487, -21.9203) -> (-25.7878, -22.9594)
  line L211 (-25.7878, -22.9594) -> (-32, -22.9594)
  line L212 (-32, -22.9594) -> (-34.0154, -24.9748)
  line L213 (-34.0154, -24.9748) -> (-27.8032, -24.9748)
  line L214 (-27.8032, -24.9748) -> (-29.8284, -27)
  line L215 (-29.8284, -27) -> (-37, -27)
  line L216 (-37, -27) -> (-40, -29.5459)
  line L217 (-40, -29.5459) -> (-32.3743, -29.5459)
  line L218 (-32.3743, -29.5459) -> (-35.7705, -32.942)
  line L219 (-35.7705, -32.942) -> (-38.9345, -32.942)
  line L220 (-38.9345, -32.942) -> (-40, -35.0405)
  line L221 (-40, -35.0405) -> (-37.8689, -35.0405)
  line L222 (-37.8689, -35.0405) -> (-40, -37.1716)
  line L223 (-40, -37.1716) -> (-40, -40)
  circle A0 centre (0, -38) radius 1
  line L224 (0, 0) -> (1.5, 0)
  line L225 (1.5, 0) -> (-1.5, 0)
  line L226 (-1.5, 0) -> (-1.5, 40)
  line L227 (-1.5, 40) -> (1.5, 40)
  line L228 (1.5, 40) -> (1.5, 0)
  dimension "d30" = 1.5
  dimension "d31" = 3
  dimension "d32" = 40
  constraint coincident L224.start origin
  constraint horizontal L224
  constraint horizontal L225
  constraint vertical L226
  constraint horizontal L227
  constraint vertical L228
  measures "d30" distance of L224.start L224.end
  measures "d31" distance of L224.end L225.end
  measures "d32" distance of L224.end L227.end
copy_body "CopyPasteBodies1" bodies 1 makes body 2
move_body "Move1" bodies 2 to x (1, 0, 0) y (0, 1, 0) z (0, 0, 1) at (113.0192, 0, 0)
extrude "Extrude2" cut sketch "Sketch4" against normal blind 3 contours L157 L158 L224 L225 L226 L228 | A0 bodies 1
sketch "Sketch5" plane through (0, 3, 0) normal (0, 1, 0) x (-1, 0, 0)
  line L0 (-121.3616, 5.514) -> (-125.9535, 5.3576)
  line L1 (-125.9535, 5.3576) -> (-122.8171, 2)
  line L2 (-122.8171, 2) -> (-137.9182, 2)
  line L3 (-137.9182, 2) -> (-131.0154, 7.4559)
  line L4 (-131.0154, 7.4559) -> (-132.0544, 16.2068)
  line L5 (-132.0544, 16.2068) -> (-121.3616, 5.514)
  line L6 (-107.5052, 8.3424) -> (-107.6616, 12.9343)
  line L7 (-107.6616, 12.9343) -> (-111.0192, 9.798)
  line L8 (-111.0192, 9.798) -> (-111.0192, 24.899)
  line L9 (-111.0192, 24.899) -> (-105.5633, 17.9962)
  line L10 (-105.5633, 17.9962) -> (-96.8124, 19.0352)
  line L11 (-96.8124, 19.0352) -> (-107.5052, 8.3424)
  line L12 (-115.0192, 9.798) -> (-118.3767, 12.9343)
  line L13 (-118.3767, 12.9343) -> (-118.5332, 8.3424)
  line L14 (-118.5332, 8.3424) -> (-129.226, 19.0352)
  line L15 (-129.226, 19.0352) -> (-120.475, 17.9962)
  line L16 (-120.475, 17.9962) -> (-115.0192, 24.899)
  line L17 (-115.0192, 24.899) -> (-115.0192, 9.798)
  line L18 (-111.0192, -9.798) -> (-107.6616, -12.9343)
  line L19 (-107.6616, -12.9343) -> (-107.5052, -8.3424)
  line L20 (-107.5052, -8.3424) -> (-96.8124, -19.0352)
  line L21 (-96.8124, -19.0352) -> (-105.5633, -17.9962)
  line L22 (-105.5633, -17.9962) -> (-111.0192, -24.899)
  line L23 (-111.0192, -24.899) -> (-111.0192, -9.798)
  line L24 (-103.2212, 2) -> (-100.0849, 5.3576)
  line L25 (-100.0849, 5.3576) -> (-104.6768, 5.514)
  line L26 (-104.6768, 5.514) -> (-93.984, 16.2068)
  line L27 (-93.984, 16.2068) -> (-95.0229, 7.4559)
  line L28 (-95.0229, 7.4559) -> (-88.1202, 2)
  line L29 (-88.1202, 2) -> (-103.2212, 2)
  line L30 (-118.5332, -8.3424) -> (-118.3767, -12.9343)
  line L31 (-118.3767, -12.9343) -> (-115.0192, -9.798)
  line L32 (-115.0192, -9.798) -> (-115.0192, -24.899)
  line L33 (-115.0192, -24.899) -> (-120.475, -17.9962)
  line L34 (-120.475, -17.9962) -> (-129.226, -19.0352)
  line L35 (-129.226, -19.0352) -> (-118.5332, -8.3424)
  line L36 (-122.8171, -2) -> (-125.9535, -5.3576)
  line L37 (-125.9535, -5.3576) -> (-121.3616, -5.514)
  line L38 (-121.3616, -5.514) -> (-132.0544, -16.2068)
  line L39 (-132.0544, -16.2068) -> (-131.0154, -7.4559)
  line L40 (-131.0154, -7.4559) -> (-137.9182, -2)
  line L41 (-137.9182, -2) -> (-122.8171, -2)
  line L42 (-95.0229, -7.4559) -> (-93.984, -16.2068)
  line L43 (-93.984, -16.2068) -> (-104.6768, -5.514)
  line L44 (-104.6768, -5.514) -> (-100.0849, -5.3576)
  line L45 (-100.0849, -5.3576) -> (-103.2212, -2)
  line L46 (-103.2212, -2) -> (-88.1202, -2)
  line L47 (-88.1202, -2) -> (-95.0229, -7.4559)
  line L48 (-153.0192, -40) -> (-150.1908, -40)
  line L49 (-150.1908, -40) -> (-148.0292, -37.8385)
  line L50 (-148.0292, -37.8385) -> (-148.0292, -40)
  line L51 (-148.0292, -40) -> (-145.9827, -38.9192)
  line L52 (-145.9827, -38.9192) -> (-145.9827, -35.792)
  line L53 (-145.9827, -35.792) -> (-142.5651, -32.3743)
  line L54 (-142.5651, -32.3743) -> (-142.5651, -40)
  line L55 (-142.5651, -40) -> (-140.0192, -37)
  line L56 (-140.0192, -37) -> (-140.0192, -29.8284)
  line L57 (-140.0192, -29.8284) -> (-138.0089, -27.8181)
  line L58 (-138.0089, -27.8181) -> (-138.0089, -33.9907)
  line L59 (-138.0089, -33.9907) -> (-136.0182, -32)
  line L60 (-136.0182, -32) -> (-136.0182, -25.8274)
  line L61 (-136.0182, -25.8274) -> (-134.9394, -24.7487)
  line L62 (-134.9394, -24.7487) -> (-122.6632, -23.2912)
  line L63 (-122.6632, -23.2912) -> (-115.0192, -32.9624)
  line L64 (-115.0192, -32.9624) -> (-115.0192, -33.9927)
  line L65 (-115.0192, -33.9927) -> (-121.0192, -40)
  line L66 (-121.0192, -40) -> (-118.0155, -40)
  line L67 (-118.0155, -40) -> (-115.0192, -37)
  line L68 (-115.0192, -37) -> (-115.0192, -38)
  line L69 (-115.0192, -38) -> (-113.0167, -40)
  line L70 (-113.0167, -40) -> (-111.0192, -38)
  line L71 (-111.0192, -38) -> (-111.0192, -36.9767)
  line L72 (-111.0192, -36.9767) -> (-107.9921, -40)
  line L73 (-107.9921, -40) -> (-105.0744, -40)
  line L74 (-105.0744, -40) -> (-111.0192, -34.0624)
  line L75 (-111.0192, -34.0624) -> (-111.0192, -32.9624)
  line L76 (-111.0192, -32.9624) -> (-103.3752, -23.2912)
  line L77 (-103.3752, -23.2912) -> (-91.0989, -24.7487)
  line L78 (-91.0989, -24.7487) -> (-90.0202, -25.8274)
  line L79 (-90.0202, -25.8274) -> (-90.0202, -32)
  line L80 (-90.0202, -32) -> (-88.0295, -33.9907)
  line L81 (-88.0295, -33.9907) -> (-88.0295, -27.8181)
  line L82 (-88.0295, -27.8181) -> (-86.0192, -29.8284)
  line L83 (-86.0192, -29.8284) -> (-86.0192, -37)
  line L84 (-86.0192, -37) -> (-83.4733, -40)
  line L85 (-83.4733, -40) -> (-83.4733, -32.3743)
  line L86 (-83.4733, -32.3743) -> (-80.0556, -35.792)
  line L87 (-80.0556, -35.792) -> (-80.0556, -38.9192)
  line L88 (-80.0556, -38.9192) -> (-78.0091, -40)
  line L89 (-78.0091, -40) -> (-78.0091, -37.8385)
  line L90 (-78.0091, -37.8385) -> (-75.8476, -40)
  line L91 (-75.8476, -40) -> (-73.0192, -40)
  line L92 (-73.0192, -40) -> (-73.0192, -37.1716)
  line L93 (-73.0192, -37.1716) -> (-75.1503, -35.0405)
  line L94 (-75.1503, -35.0405) -> (-73.0192, -35.0405)
  line L95 (-73.0192, -35.0405) -> (-74.0847, -32.942)
  line L96 (-74.0847, -32.942) -> (-77.2487, -32.942)
  line L97 (-77.2487, -32.942) -> (-80.6448, -29.5459)
  line L98 (-80.6448, -29.5459) -> (-73.0192, -29.5459)
  line L99 (-73.0192, -29.5459) -> (-76.0192, -27)
  line L100 (-76.0192, -27) -> (-83.1908, -27)
  line L101 (-83.1908, -27) -> (-85.2159, -24.9748)
  line L102 (-85.2159, -24.9748) -> (-79.0037, -24.9748)
  line L103 (-79.0037, -24.9748) -> (-81.0192, -22.9594)
  line L104 (-81.0192, -22.9594) -> (-87.2314, -22.9594)
  line L105 (-87.2314, -22.9594) -> (-88.2705, -21.9203)
  line L106 (-88.2705, -21.9203) -> (-89.728, -9.644)
  line L107 (-89.728, -9.644) -> (-80.0568, -2)
  line L108 (-80.0568, -2) -> (-79.0192, -2)
  line L109 (-79.0192, -2) -> (-73.0192, -8)
  line L110 (-73.0192, -8) -> (-73.0192, -5)
  line L111 (-73.0192, -5) -> (-76.0192, -2)
  line L112 (-76.0192, -2) -> (-75.0192, -2)
  line L113 (-75.0192, -2) -> (-73.0192, 0)
  line L114 (-73.0192, 0) -> (-75.0192, 2)
  line L115 (-75.0192, 2) -> (-76.0192, 2)
  line L116 (-76.0192, 2) -> (-73.0192, 5)
  line L117 (-73.0192, 5) -> (-73.0192, 8)
  line L118 (-73.0192, 8) -> (-79.0192, 2)
  line L119 (-79.0192, 2) -> (-80.0568, 2)
  line L120 (-80.0568, 2) -> (-89.728, 9.644)
  line L121 (-89.728, 9.644) -> (-88.2705, 21.9203)
  line L122 (-88.2705, 21.9203) -> (-87.2314, 22.9594)
  line L123 (-87.2314, 22.9594) -> (-81.0192, 22.9594)
  line L124 (-81.0192, 22.9594) -> (-79.0037, 24.9748)
  line L125 (-79.0037, 24.9748) -> (-85.2159, 24.9748)
  line L126 (-85.2159, 24.9748) -> (-83.1908, 27)
  line L127 (-83.1908, 27) -> (-76.0192, 27)
  line L128 (-76.0192, 27) -> (-73.0192, 29.5459)
  line L129 (-73.0192, 29.5459) -> (-80.6448, 29.5459)
  line L130 (-80.6448, 29.5459) -> (-77.2487, 32.942)
  line L131 (-77.2487, 32.942) -> (-74.0847, 32.942)
  line L132 (-74.0847, 32.942) -> (-73.0192, 35.0405)
  line L133 (-73.0192, 35.0405) -> (-75.1503, 35.0405)
  line L134 (-75.1503, 35.0405) -> (-73.0192, 37.1716)
  line L135 (-73.0192, 37.1716) -> (-73.0192, 40)
  line L136 (-73.0192, 40) -> (-75.8476, 40)
  line L137 (-75.8476, 40) -> (-78.0091, 37.8385)
  line L138 (-78.0091, 37.8385) -> (-78.0091, 40)
  line L139 (-78.0091, 40) -> (-80.0556, 38.9192)
  line L140 (-80.0556, 38.9192) -> (-80.0556, 35.792)
  line L141 (-80.0556, 35.792) -> (-83.4733, 32.3743)
  line L142 (-83.4733, 32.3743) -> (-83.4733, 40)
  line L143 (-83.4733, 40) -> (-86.0192, 37)
  line L144 (-86.0192, 37) -> (-86.0192, 29.8284)
  line L145 (-86.0192, 29.8284) -> (-88.0295, 27.8181)
  line L146 (-88.0295, 27.8181) -> (-88.0295, 33.9907)
  line L147 (-88.0295, 33.9907) -> (-90.0202, 32)
  line L148 (-90.0202, 32) -> (-90.0202, 25.8274)
  line L149 (-90.0202, 25.8274) -> (-91.0989, 24.7487)
  line L150 (-91.0989, 24.7487) -> (-103.3752, 23.2912)
  line L151 (-103.3752, 23.2912) -> (-111.0192, 32.9624)
  line L152 (-111.0192, 32.9624) -> (-111.0192, 34.0088)
  line L153 (-111.0192, 34.0088) -> (-105.028, 40)
  line L154 (-105.028, 40) -> (-108.0168, 40)
  line L155 (-108.0168, 40) -> (-111.0192, 36.9976)
  line L156 (-111.0192, 36.9976) -> (-111.0192, 38)
  line L157 (-111.0192, 38) -> (-113.0192, 40)
  line L158 (-113.0192, 40) -> (-115.0192, 38)
  line L159 (-115.0192, 38) -> (-115.0192, 37.0044)
  line L160 (-115.0192, 37.0044) -> (-118.0148, 40)
  line L161 (-118.0148, 40) -> (-121.0103, 40)
  line L162 (-121.0103, 40) -> (-115.0192, 34.0088)
  line L163 (-115.0192, 34.0088) -> (-115.0192, 32.9624)
  line L164 (-115.0192, 32.9624) -> (-122.6632, 23.2912)
  line L165 (-122.6632, 23.2912) -> (-134.9394, 24.7487)
  line L166 (-134.9394, 24.7487) -> (-136.0182, 25.8274)
  line L167 (-136.0182, 25.8274) -> (-136.0182, 32)
  line L168 (-136.0182, 32) -> (-138.0089, 33.9907)
  line L169 (-138.0089, 33.9907) -> (-138.0089, 27.8181)
  line L170 (-138.0089, 27.8181) -> (-140.0192, 29.8284)
  line L171 (-140.0192, 29.8284) -> (-140.0192, 37)
  line L172 (-140.0192, 37) -> (-142.5651, 40)
  line L173 (-142.5651, 40) -> (-142.5651, 32.3743)
  line L174 (-142.5651, 32.3743) -> (-145.9827, 35.792)
  line L175 (-145.9827, 35.792) -> (-145.9827, 38.9192)
  line L176 (-145.9827, 38.9192) -> (-148.0292, 40)
  line L177 (-148.0292, 40) -> (-148.0292, 37.8385)
  line L178 (-148.0292, 37.8385) -> (-150.1908, 40)
  line L179 (-150.1908, 40) -> (-153.0192, 40)
  line L180 (-153.0192, 40) -> (-153.0192, 37.1716)
  line L181 (-153.0192, 37.1716) -> (-150.8881, 35.0405)
  line L182 (-150.8881, 35.0405) -> (-153.0192, 35.0405)
  line L183 (-153.0192, 35.0405) -> (-151.9536, 32.942)
  line L184 (-151.9536, 32.942) -> (-148.7897, 32.942)
  line L185 (-148.7897, 32.942) -> (-145.3935, 29.5459)
  line L186 (-145.3935, 29.5459) -> (-153.0192, 29.5459)
  line L187 (-153.0192, 29.5459) -> (-150.0192, 27)
  line L188 (-150.0192, 27) -> (-142.8476, 27)
  line L189 (-142.8476, 27) -> (-140.8224, 24.9748)
  line L190 (-140.8224, 24.9748) -> (-147.0346, 24.9748)
  line L191 (-147.0346, 24.9748) -> (-145.0192, 22.9594)
  line L192 (-145.0192, 22.9594) -> (-138.807, 22.9594)
  line L193 (-138.807, 22.9594) -> (-137.7679, 21.9203)
  line L194 (-137.7679, 21.9203) -> (-136.3103, 9.644)
  line L195 (-136.3103, 9.644) -> (-145.9815, 2)
  line L196 (-145.9815, 2) -> (-147.0078, 2)
  line L197 (-147.0078, 2) -> (-153.0192, 8)
  line L198 (-153.0192, 8) -> (-153.0192, 4.9575)
  line L199 (-153.0192, 4.9575) -> (-150.0561, 2)
  line L200 (-150.0561, 2) -> (-151.023, 2)
  line L201 (-151.023, 2) -> (-153.0192, 0)
  line L202 (-153.0192, 0) -> (-151.0154, -2)
  line L203 (-151.0154, -2) -> (-150.0561, -2)
  line L204 (-150.0561, -2) -> (-153.0192, -4.9687)
  line L205 (-153.0192, -4.9687) -> (-153.0192, -7.9488)
  line L206 (-153.0192, -7.9488) -> (-147.0816, -2)
  line L207 (-147.0816, -2) -> (-145.9815, -2)
  line L208 (-145.9815, -2) -> (-136.3103, -9.644)
  line L209 (-136.3103, -9.644) -> (-137.7679, -21.9203)
  line L210 (-137.7679, -21.9203) -> (-138.807, -22.9594)
  line L211 (-138.807, -22.9594) -> (-145.0192, -22.9594)
  line L212 (-145.0192, -22.9594) -> (-147.0346, -24.9748)
  line L213 (-147.0346, -24.9748) -> (-140.8224, -24.9748)
  line L214 (-140.8224, -24.9748) -> (-142.8476, -27)
  line L215 (-142.8476, -27) -> (-150.0192, -27)
  line L216 (-150.0192, -27) -> (-153.0192, -29.5459)
  line L217 (-153.0192, -29.5459) -> (-145.3935, -29.5459)
  line L218 (-145.3935, -29.5459) -> (-148.7897, -32.942)
  line L219 (-148.7897, -32.942) -> (-151.9536, -32.942)
  line L220 (-151.9536, -32.942) -> (-153.0192, -35.0405)
  line L221 (-153.0192, -35.0405) -> (-150.8881, -35.0405)
  line L222 (-150.8881, -35.0405) -> (-153.0192, -37.1716)
  line L223 (-153.0192, -37.1716) -> (-153.0192, -40)
  line L224 (-113, 0) -> (-111.5, 0)
  line L225 (-111.5, 0) -> (-114.5, 0)
  line L226 (-111.5, 0) -> (-114.5, 0)
  line L227 (-114.5, 0) -> (-114.5, -40)
  line L228 (-114.5, -40) -> (-111.5, -40)
  line L229 (-111.5, -40) -> (-111.5, 0)
  dimension "d40" = 1.5
  dimension "d41" = 3
  dimension "d42" = 40
  constraint horizontal L224
  constraint parallel L224 L225
  constraint horizontal L226
  constraint vertical L227
  constraint horizontal L228
  constraint vertical L229
  measures "d40" distance of L224.start L224.end
  measures "d41" distance of L224.end L225.end
  measures "d42" distance of L224.end L228.end
extrude "Extrude4" cut sketch "Sketch5" against normal blind 3 contours L69 L70 L224 L225 L226 L227 L229 bodies 2
